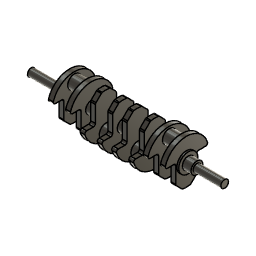
Crankshaft_ (Autodesk Fusion 360 design; units mm, degrees)
Autodesk Fusion 360 part; units mm, degrees
sketch "Sketch1" plane through (0, 0, 0) normal (0, 1, 0) x (1, 0, 0)
  line L0 (0, 0) -> (1016, 0)
  line L1 (1016, 0) -> (1016, -254)
  line L2 (1016, -254) -> (965.2, -254)
  line L3 (965.2, -254) -> (965.2, -158.75)
  line L4 (965.2, -158.75) -> (736.6, -158.75)
  line L5 (736.6, -158.75) -> (736.6, -101.6)
  line L6 (736.6, -101.6) -> (0, -101.6)
  line L7 (0, -101.6) -> (0, 0)
  dimension "d1" = 1016
  dimension "d2" = 203.2
  dimension "d3" = 317.5
  dimension "d4" = 508
  dimension "d5" = 50.8
  dimension "d6" = 228.6
  constraint coincident L0.start L7.end
  constraint horizontal L0
  constraint perpendicular L0 L1
  constraint perpendicular L1 L2
  constraint perpendicular L2 L3
  constraint perpendicular L3 L4
  constraint perpendicular L4 L5
  constraint perpendicular L5 L6
  constraint perpendicular L0 L7
  measures "d1" distance of L0.start L0.end
  measures "d5" distance of L1.end L2.end
  measures "d6" distance of L3.end L4.end
revolve "Revolve1" add sketch "Sketch1" angle 360 about axis through (0, 0, 0) along (1, 0, 0)
sketch "Sketch2" plane through (1016, 0, 0) normal (1, 0, 0) x (0, 1, 0)
  circle A0 centre (0, 0) radius 254
  line L0 (-575.2974, 101.6) -> (-279.4, 101.6)
  line L1 (-279.4, 101.6) -> (-279.4, -406.4)
  line L2 (-279.4, -406.4) -> (-112.5429, -573.2571)
  line L3 (0, 0) -> (0, -701.9351) construction
  line L4 (279.4, -406.4) -> (112.5429, -573.2571)
  line L5 (279.4, 101.6) -> (279.4, -406.4)
  line L6 (575.2974, 101.6) -> (279.4, 101.6)
  arc A1 (575.2974, 101.6) -> (-575.2974, 101.6) centre (0, 0) ccw
  arc A2 (-112.5429, -573.2571) -> (112.5429, -573.2571) centre (0, 0) ccw
  dimension "d8" = 1168.4
  dimension "d9" = 101.6
  dimension "d10" = 135
  dimension "d11" = 508
  dimension "d12" = 558.8
  constraint concentric A0 A1
  constraint horizontal L0
  constraint perpendicular L0 L1
  constraint coincident L2.end A1
  constraint coincident A0.centre L3.start
  constraint vertical L3
  constraint symmetric L0.start L3 L6.start
  constraint symmetric L0.end L3 L5.start
  constraint symmetric L1.end L3 L4.start
  constraint symmetric L2.end L3 L4.end
  constraint concentric A1 A2
  measures "d8" diameter of A1
  measures "d9" distance of A0.centre L0
  measures "d10" angle of L1 L2
  measures "d11" distance of L0.end L1.end
  measures "d12" distance of L1 L5
extrude "Extrude1" add sketch "Sketch2" along normal blind 127 contours A0 | L0 L1 L2 L4 L5 L6 A1 A2
fillet "Fillet1" radius 50.8 8 edges at (1079.5, 575.2974, 101.6) (1079.5, 279.4, 101.6) (1079.5, 279.4, -406.4) (1079.5, 112.5429, -573.2571) (1079.5, -112.5429, -573.2571) (1079.5, -279.4, -406.4) (1079.5, -279.4, 101.6) (1079.5, -575.2974, 101.6)
sketch "Sketch3" plane through (1143, 0, 0) normal (1, 0, 0) x (0, 1, 0)
  arc A0 (-559.8475, 166.9143) -> (-511.1651, 101.6) centre (-511.1651, 152.4) ccw
  line L0 (-511.1651, 101.6) -> (-330.2, 101.6)
  arc A1 (-279.4, 50.8) -> (-330.2, 101.6) centre (-330.2, 50.8) ccw
  line L1 (-279.4, 50.8) -> (-279.4, -385.358)
  arc A2 (-279.4, -385.358) -> (-264.521, -421.279) centre (-228.6, -385.358) ccw
  line L2 (-264.521, -421.279) -> (-123.7615, -562.0385)
  arc A3 (-123.7615, -562.0385) -> (-96.2062, -576.2239) centre (-87.8405, -526.1175) ccw
  arc A4 (-96.2062, -576.2239) -> (96.2062, -576.2239) centre (0, 0) ccw
  arc A5 (96.2062, -576.2239) -> (123.7615, -562.0385) centre (87.8405, -526.1175) ccw
  line L3 (123.7615, -562.0385) -> (264.521, -421.279)
  arc A6 (264.521, -421.279) -> (279.4, -385.358) centre (228.6, -385.358) ccw
  line L4 (279.4, -385.358) -> (279.4, 50.8)
  arc A7 (330.2, 101.6) -> (279.4, 50.8) centre (330.2, 50.8) ccw
  line L5 (330.2, 101.6) -> (511.1651, 101.6)
  arc A8 (511.1651, 101.6) -> (559.8475, 166.9143) centre (511.1651, 152.4) ccw
  arc A9 (559.8475, 166.9143) -> (-559.8475, 166.9143) centre (0, 0) ccw
  circle A10 centre (0, 355.6) radius 177.8
  dimension "d17" = 355.6
  dimension "d18" = 355.6
  constraint vertical A4.centre A10.centre
  measures "d17" diameter of A10
  measures "d18" distance of A4.centre A10.centre
extrude "Extrude2" add sketch "Sketch3" along normal blind 330.2 contours A10
pattern_linear "R-Pattern1" count 2 spacing 457.2 along (1, 0, 0) of "Extrude1", "Fillet1"
sketch "Sketch4" plane through (1600.2, 0, 0) normal (1, 0, 0) x (0, 1, 0)
  arc A0 (-559.8475, 166.9143) -> (-511.1651, 101.6) centre (-511.1651, 152.4) ccw
  line L0 (-511.1651, 101.6) -> (-330.2, 101.6)
  arc A1 (-279.4, 50.8) -> (-330.2, 101.6) centre (-330.2, 50.8) ccw
  line L1 (-279.4, 50.8) -> (-279.4, -385.358)
  arc A2 (-279.4, -385.358) -> (-264.521, -421.279) centre (-228.6, -385.358) ccw
  line L2 (-264.521, -421.279) -> (-123.7615, -562.0385)
  arc A3 (-123.7615, -562.0385) -> (-96.2062, -576.2239) centre (-87.8405, -526.1175) ccw
  arc A4 (-96.2062, -576.2239) -> (96.2062, -576.2239) centre (0, 0) ccw
  arc A5 (96.2062, -576.2239) -> (123.7615, -562.0385) centre (87.8405, -526.1175) ccw
  line L3 (123.7615, -562.0385) -> (264.521, -421.279)
  arc A6 (264.521, -421.279) -> (279.4, -385.358) centre (228.6, -385.358) ccw
  line L4 (279.4, -385.358) -> (279.4, 50.8)
  arc A7 (330.2, 101.6) -> (279.4, 50.8) centre (330.2, 50.8) ccw
  line L5 (330.2, 101.6) -> (511.1651, 101.6)
  arc A8 (511.1651, 101.6) -> (559.8475, 166.9143) centre (511.1651, 152.4) ccw
  arc A9 (559.8475, 166.9143) -> (-559.8475, 166.9143) centre (0, 0) ccw
  circle A10 centre (0, 0) radius 158.75
  dimension "d25" = 317.5
  constraint coincident A4.centre A9.centre
  measures "d25" diameter of A10
extrude "Extrude3" add sketch "Sketch4" along normal blind 254 contours A10
sketch "Sketch5" plane through (1854.2, 0, 0) normal (1, 0, 0) x (0, 1, 0)
  circle A0 centre (0, 0) radius 158.75
  line L0 (-575.2974, -101.6) -> (-279.4, -101.6)
  line L1 (-279.4, -101.6) -> (-279.4, 406.4)
  line L2 (-279.4, 406.4) -> (-112.5429, 573.2571)
  line L3 (0, 0) -> (0, 823.9979) construction
  line L4 (575.2974, -101.6) -> (279.4, -101.6)
  line L5 (279.4, -101.6) -> (279.4, 406.4)
  line L6 (279.4, 406.4) -> (112.5429, 573.2571)
  arc A1 (-575.2974, -101.6) -> (575.2974, -101.6) centre (0, 0) ccw
  arc A2 (112.5429, 573.2571) -> (-112.5429, 573.2571) centre (0, 0) ccw
  dimension "d28" = 1168.4
  dimension "d29" = 135
  dimension "d30" = 508
  dimension "d31" = 279.4
  dimension "d32" = 101.6
  dimension "d33" = 584.2
  constraint concentric A0 A1
  constraint horizontal L0
  constraint perpendicular L0 L1
  constraint coincident A0.centre L3.start
  constraint parallel L1 L3
  constraint symmetric L0.start L3 L4.start
  constraint symmetric L0.end L3 L4.end
  constraint symmetric L1.end L3 L5.end
  constraint symmetric L2.end L3 L6.end
  constraint concentric A1 A2
  measures "d28" diameter of A1
  measures "d29" angle of L1 L2
  measures "d30" distance of L0.end L1.end
  measures "d31" distance of L1 L3
  measures "d32" distance of A0.centre L0
  measures "d33" radius of A2
extrude "Extrude4" add sketch "Sketch5" along normal blind 127 contours A0 | L0 L1 L2 L4 L5 L6 A1 A2
fillet "Fillet2" radius 50.8 8 edges at (1917.7, -279.4, -101.6) (1917.7, -575.2974, -101.6) (1917.7, -279.4, 406.4) (1917.7, -112.5429, 573.2571) (1917.7, 112.5429, 573.2571) (1917.7, 279.4, 406.4) (1917.7, 279.4, -101.6) (1917.7, 575.2974, -101.6)
sketch "Sketch6" plane through (1981.2, 0, 0) normal (1, 0, 0) x (0, 1, 0)
  arc A0 (559.8475, -166.9143) -> (511.1651, -101.6) centre (511.1651, -152.4) ccw
  line L0 (511.1651, -101.6) -> (330.2, -101.6)
  arc A1 (279.4, -50.8) -> (330.2, -101.6) centre (330.2, -50.8) ccw
  line L1 (279.4, -50.8) -> (279.4, 385.358)
  arc A2 (279.4, 385.358) -> (264.521, 421.279) centre (228.6, 385.358) ccw
  line L2 (264.521, 421.279) -> (123.7615, 562.0385)
  arc A3 (123.7615, 562.0385) -> (96.2062, 576.2239) centre (87.8405, 526.1175) ccw
  arc A4 (96.2062, 576.2239) -> (-96.2062, 576.2239) centre (0, 0) ccw
  arc A5 (-96.2062, 576.2239) -> (-123.7615, 562.0385) centre (-87.8405, 526.1175) ccw
  line L3 (-123.7615, 562.0385) -> (-264.521, 421.279)
  arc A6 (-264.521, 421.279) -> (-279.4, 385.358) centre (-228.6, 385.358) ccw
  line L4 (-279.4, 385.358) -> (-279.4, -50.8)
  arc A7 (-330.2, -101.6) -> (-279.4, -50.8) centre (-330.2, -50.8) ccw
  line L5 (-330.2, -101.6) -> (-511.1651, -101.6)
  arc A8 (-511.1651, -101.6) -> (-559.8475, -166.9143) centre (-511.1651, -152.4) ccw
  arc A9 (-559.8475, -166.9143) -> (559.8475, -166.9143) centre (0, 0) ccw
  circle A10 centre (0, -355.6) radius 177.8
  dimension "d38" = 355.6
  dimension "d39" = 355.6
  constraint vertical A4.centre A10.centre
  measures "d38" diameter of A10
  measures "d39" distance of A4.centre A10.centre
extrude "Extrude5" add sketch "Sketch6" along normal blind 330.2 contours A10
pattern_linear "R-Pattern2" count 2 spacing 457.2 along (1, 0, 0) of "Extrude4", "Fillet2"
sketch "Sketch7" plane through (2438.4, 0, 0) normal (1, 0, 0) x (0, 1, 0)
  arc A0 (559.8475, -166.9143) -> (511.1651, -101.6) centre (511.1651, -152.4) ccw
  line L0 (511.1651, -101.6) -> (330.2, -101.6)
  arc A1 (279.4, -50.8) -> (330.2, -101.6) centre (330.2, -50.8) ccw
  line L1 (279.4, -50.8) -> (279.4, 385.358)
  arc A2 (279.4, 385.358) -> (264.521, 421.279) centre (228.6, 385.358) ccw
  line L2 (264.521, 421.279) -> (123.7615, 562.0385)
  arc A3 (123.7615, 562.0385) -> (96.2062, 576.2239) centre (87.8405, 526.1175) ccw
  arc A4 (96.2062, 576.2239) -> (-96.2062, 576.2239) centre (0, 0) ccw
  arc A5 (-96.2062, 576.2239) -> (-123.7615, 562.0385) centre (-87.8405, 526.1175) ccw
  line L3 (-123.7615, 562.0385) -> (-264.521, 421.279)
  arc A6 (-264.521, 421.279) -> (-279.4, 385.358) centre (-228.6, 385.358) ccw
  line L4 (-279.4, 385.358) -> (-279.4, -50.8)
  arc A7 (-330.2, -101.6) -> (-279.4, -50.8) centre (-330.2, -50.8) ccw
  line L5 (-330.2, -101.6) -> (-511.1651, -101.6)
  arc A8 (-511.1651, -101.6) -> (-559.8475, -166.9143) centre (-511.1651, -152.4) ccw
  arc A9 (-559.8475, -166.9143) -> (559.8475, -166.9143) centre (0, 0) ccw
  circle A10 centre (0, 0) radius 158.75
  dimension "d46" = 317.5
  constraint coincident A4.centre A9.centre
  measures "d46" diameter of A10
extrude "Extrude6" add sketch "Sketch7" along normal blind 127 contours A10
mirror "Mirror1" about plane through (2565.4, 0, 0) normal (1, 0, 0) of bodies 1 merged
